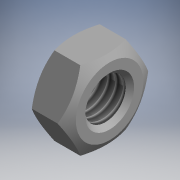
# Autodesk Inventor part: NTJ-015C
Saved by Autodesk Inventor 2017.3 (Build 213256000, 256)
## iProperties
Part Number: NTJ-015C
Material: Generic
Catalog Web Link: www.cadenas.de
Description: CJ2-Z_NTJ-Rod End Nut
Vendor: SMC
Document SubType Name: Modeling
Designer: partserver
Manufacturer: SMC
Mass: 0.156621 g
Surface Area: 2.21641 cm^2
Volume: 0.156621 cm^3
Density: 1 g/cm^3
Appearance: PSOLRGB-191-191-191
Category: PARTsolutions
Company: SMC
Title: NTJ-015C
Author: Cadenas PARTsolutions
Comments: Rod End Nut
PSOL_IDENT_0: {$CADENAS_DATA\23d-libs\smc_jp\actuator\standard_air_cylinder\cj2\accessories\cj2_z_ntj.prj},159 {VT
PSOL_IDENT_1: YP=3D},{NB=NTJ-015C},{LINA=NTJ-015C},{NN=CJ2-Z_NTJ},{DATE=29.10.2021 06:22:47},{GEOMDATE=26.04.2020
PSOL_IDENT_2: 07:35:34},{VERSION=},{LINEID=30},{WBVAR=},{WBNUMERIC=}  {NB=NTJ-015C},{LINA=NTJ-015C},{KT=DUMMY},{MO
PSOL_IDENT_3: DEL=NTJ-015C},{BORE=16},{B2=8.0},{C2=9.2},{D=M5x0.8},{D1=5},{D2=0.8},{H2=4.0},{DW=6.88},{ORDER=NTJ-0
PSOL_IDENT_4: 15C}
NB: NTJ-015C
NN: CJ2-Z_NTJ
NT: Rod End Nut
NBSYN: $MODEL.
LINA: NTJ-015C
CATALOG: SMC (JP
MODEL: NTJ-015C
BORE: 16
SUPPLIER: SMC
ARTICLENO: NTJ-015C
BOMINFO: NTJ-015C
CREATOR: CADENAS GmbH
Autodesk Inventor part; units mm, degrees
sketch "B" plane through (0, 0, 0) normal (1, 0, 0) x (0, 1, 0)
  line L0 (-2.3094, 4) -> (-4.6188, 0)
  line L1 (-4.6188, 0) -> (-2.3094, -4)
  line L2 (-2.3094, -4) -> (2.3094, -4)
  line L3 (2.3094, -4) -> (4.6188, 0)
  line L4 (4.6188, 0) -> (2.3094, 4)
  line L5 (2.3094, 4) -> (-2.3094, 4)
  constraints: 12 end point
extrude "Extrusion1" add sketch "B" along normal mid plane 4
sketch "Sketch_2" plane through (0, 0, 0) normal (0, 0, 1) x (1, 0, 0)
  line L0 (2, 0) -> (-2, 0)
  line L1 (-2, 0) -> (-2, 2.5)
  line L2 (-2, 2.5) -> (-1.567, 2.067)
  line L3 (-1.567, 2.067) -> (1.567, 2.067)
  line L4 (1.567, 2.067) -> (2, 2.5)
  line L5 (2, 2.5) -> (2, 0)
  line L6 (2, 0) -> (-2, 0)
  constraints: 14 end point
revolve "Revolution1" cut sketch "Sketch_2" angle 360 about axis through (2, 0, 0) along (1, 0, 0)
thread "Thread1" size "M5x0.8" class "6H" standard "ISO Metric profile" full length
sketch "Sketch_3" plane through (0, 0, 0) normal (0, 0, 1) x (1, 0, 0)
  line L0 (50, 0) -> (-50, 0)
  line L1 (-7, 1) -> (-2, 1)
  line L2 (-2, 1) -> (-2, 3.44)
  line L3 (-2, 3.44) -> (0, 6.9041)
  line L4 (0, 6.9041) -> (2, 3.44)
  line L5 (2, 3.44) -> (2, 1)
  line L6 (2, 1) -> (7, 1)
  line L7 (7, 1) -> (7, 8.44)
  line L8 (7, 8.44) -> (-7, 8.44)
  line L9 (-7, 8.44) -> (-7, 1)
  constraints: 20 end point
revolve "Revolution2" cut sketch "Sketch_3" angle 360 about axis through (50, 0, 0) along (1, 0, 0)
ref_plane "nt_XY" through (0, 0, 0) normal (1, 0, 0) x (0, 0, -1)
ref_plane "nt_YZ" through (0, 0, 0) normal (0, 0, -1) x (0, 1, 0)
ref_plane "nt_ZX" through (0, 0, 0) normal (0, 1, 0) x (1, 0, 0)
ref_plane "ntj_XY" through (2, 0, 0) normal (1, 0, 0) x (0, 0, -1)
ref_plane "ntj_YZ" through (2, 0, 0) normal (0, 0, -1) x (0, 1, 0)
ref_plane "ntj_ZX" through (2, 0, 0) normal (0, 1, 0) x (1, 0, 0)
body "Solid1"
